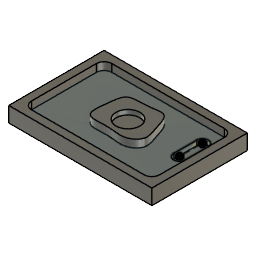
Cam Milling 1 (Autodesk Fusion 360 design; units mm, degrees)
part number: 2026-06-20-21-11-02-857
Autodesk Fusion 360 part; units mm, degrees
sketch "Sketch1" plane through (0, 0, 0) normal (0, 0, 1) x (1, 0, 0)
  line L0 (-75, 50) -> (75, 50)
  line L1 (75, 50) -> (75, -50)
  line L2 (75, -50) -> (-75, -50)
  line L3 (-75, -50) -> (-75, 50)
  line L4 (-75, 50) -> (75, -50) construction
  line L5 (75, 50) -> (-75, -50) construction
  line L6 (59, -42) -> (-59, -42)
  line L7 (-67, -34) -> (-67, 34)
  line L8 (-59, 42) -> (59, 42)
  line L9 (67, 34) -> (67, -34)
  spline S0 degree 5 poles (0, 22.4638) (-0.8512, 22.3723) (-2.5749, 22.2065) (-5.2041, 22.0186) (-8.7034, 21.8851) (-12.8111, 21.7572) (-16.4137, 21.4266) (-19.3328, 20.6302) (-21.4856, 19.1397) (-22.9396, 16.8333) (-23.8797, 13.7066) (-24.5296, 9.8513) (-25.0848, 5.4458) (-25.6462, 0.739) (-26.1388, -3.9587) (-26.3602, -8.3171) (-26.0551, -12.0321) (-24.9834, -14.8737) (-22.9846, -16.7269) (-20.0608, -17.6506) (-16.39, -17.8744) (-12.2425, -17.7077) (-7.9213, -17.4694) (-3.6953, -17.4135) (0.2717, -17.6471) (3.9677, -18.0777) (7.463, -18.4971) (10.8553, -18.6466) (14.2107, -18.2888) (17.5046, -17.2781) (20.5668, -15.6275) (23.1569, -13.4486) (25.0395, -10.8925) (26.0506, -8.0979) (26.1887, -5.1193) (25.6129, -1.9281) (24.5591, 1.5242) (23.2765, 5.2568) (21.9612, 9.2114) (20.6767, 13.1862) (19.3688, 16.8808) (17.9149, 19.9787) (16.1624, 22.2215) (13.9692, 23.4772) (11.2494, 23.8354) (7.9839, 23.5599) (4.97, 23.0978) (2.5324, 22.7554) (0.8512, 22.5553) (0, 22.4638) knots 0 0 0 0 0 0 0.022222 0.044444 0.066667 0.088889 0.111111 0.133333 0.155556 0.177778 0.2 0.222222 0.244444 0.266667 0.288889 0.311111 0.333333 0.355556 0.377778 0.4 0.422222 0.444444 0.466667 0.488889 0.511111 0.533333 0.555556 0.577778 0.6 0.622222 0.644444 0.666667 0.688889 0.711111 0.733333 0.755556 0.777778 0.8 0.822222 0.844444 0.866667 0.888889 0.911111 0.933333 0.955556 0.977778 1 1 1 1 1 1
  arc A0 (-59, 42) -> (-67, 34) centre (-59, 34) ccw
  arc A1 (67, 34) -> (59, 42) centre (59, 34) ccw
  arc A2 (59, -42) -> (67, -34) centre (59, -34) ccw
  arc A3 (-67, -34) -> (-59, -42) centre (-59, -34) ccw
  point P0 (-20, 20)
  point P1 (-25.1867, 4.5381)
  point P2 (-23.7205, -15.8137)
  point P3 (-4.5381, -17.4719)
  point P4 (14.0682, -18.1526)
  point P5 (25.4136, -9.5301)
  point P6 (22.9176, 6.3534)
  point P7 (15.4297, 22.4638)
  dimension "d1" = 100
  dimension "d2" = 150
  dimension "d9" = 8
  constraint horizontal L0
  constraint perpendicular L0 L1
  constraint parallel L0 L2
  constraint parallel L1 L3
  constraint coincident L4 origin
  constraint coincident L5 origin
  constraint coincident L5 P2
  constraint tangent L7 A0
  constraint tangent L8 A0
  constraint tangent L8 A1
  constraint tangent L9 A1
  constraint equal A0 A1
  constraint tangent L6 A2
  constraint tangent L9 A2
  constraint equal A0 A2
  constraint tangent L6 A3
  constraint tangent L7 A3
  constraint equal A0 A3
  measures "d1" distance of L0.end L1.end
  measures "d2" distance of L1 L3
  measures "d9" radius of A0
extrude "Extrude1" add sketch "Sketch1" along normal blind 8 contours L0 L1 L2 L3 | L6 L7 L8 L9 A0 A1 A2 A3 | S0 makes body 1
extrude "Extrude2" add sketch "Sketch1" along normal blind 8 from surface at 8 bodies 1
sketch "Sketch2" plane through (0, 0, 8) normal (0, 0, 1) x (-1, 0, 0)
  spline S0 degree 5 poles (0, -22.4638) (-0.8512, -22.5553) (-2.5324, -22.7554) (-4.97, -23.0978) (-7.9839, -23.5599) (-11.2494, -23.8354) (-13.9692, -23.4772) (-16.1624, -22.2215) (-17.9149, -19.9787) (-19.3688, -16.8808) (-20.6767, -13.1862) (-21.9612, -9.2114) (-23.2765, -5.2568) (-24.5591, -1.5242) (-25.6129, 1.9281) (-26.1887, 5.1193) (-26.0506, 8.0979) (-25.0395, 10.8925) (-23.1569, 13.4486) (-20.5668, 15.6275) (-17.5046, 17.2781) (-14.2107, 18.2888) (-10.8553, 18.6466) (-7.463, 18.4971) (-3.9677, 18.0777) (-0.2717, 17.6471) (3.6953, 17.4135) (7.9213, 17.4694) (12.2425, 17.7077) (16.39, 17.8744) (20.0608, 17.6506) (22.9846, 16.7269) (24.9834, 14.8737) (26.0551, 12.0321) (26.3602, 8.3171) (26.1388, 3.9587) (25.6462, -0.739) (25.0848, -5.4458) (24.5296, -9.8513) (23.8797, -13.7066) (22.9396, -16.8333) (21.4856, -19.1397) (19.3328, -20.6302) (16.4137, -21.4266) (12.8111, -21.7572) (8.7034, -21.8851) (5.2041, -22.0186) (2.5749, -22.2065) (0.8512, -22.3723) (0, -22.4638) knots -1 -1 -1 -1 -1 -1 -0.977778 -0.955556 -0.933333 -0.911111 -0.888889 -0.866667 -0.844444 -0.822222 -0.8 -0.777778 -0.755556 -0.733333 -0.711111 -0.688889 -0.666667 -0.644444 -0.622222 -0.6 -0.577778 -0.555556 -0.533333 -0.511111 -0.488889 -0.466667 -0.444444 -0.422222 -0.4 -0.377778 -0.355556 -0.333333 -0.311111 -0.288889 -0.266667 -0.244444 -0.222222 -0.2 -0.177778 -0.155556 -0.133333 -0.111111 -0.088889 -0.066667 -0.044444 -0.022222 0 0 0 0 0 0
  line L0 (67, -34) -> (67, 34)
  arc A0 (67, 34) -> (59, 42) centre (59, 34) ccw
  line L1 (59, 42) -> (-59, 42)
  arc A1 (-59, 42) -> (-67, 34) centre (-59, 34) ccw
  line L2 (-67, 34) -> (-67, -34)
  arc A2 (-67, -34) -> (-59, -42) centre (-59, -34) ccw
  line L3 (-59, -42) -> (59, -42)
  arc A3 (59, -42) -> (67, -34) centre (59, -34) ccw
  line L4 (-47, -25) -> (-47, -1)
  arc A4 (-47, -1) -> (-59, -1) centre (-53, -1) ccw
  line L5 (-59, -1) -> (-59, -25)
  arc A5 (-59, -25) -> (-47, -25) centre (-53, -25) ccw
  line L6 (-53, -25) -> (-53, -1) construction
  dimension "d10" = 24
  dimension "d11" = 6
  dimension "d12" = 14
  dimension "d13" = 17
  constraint tangent L4 A4
  constraint tangent A4 L5
  constraint parallel L4 L5
  constraint tangent L5 A5
  constraint tangent L4 A5
  constraint vertical L6
  measures "d10" distance of A5.centre A4.centre
  measures "d11" radius of A5
  measures "d12" distance of L2 L6
  measures "d13" distance of L3 A5.centre
surface "Extrude3" add extruded along (0, 0, 1) between 0 and -8 profiles "Sketch2" section 1 contours L4 A4 L5 A5 separate body makes body 2
extrude "Extrude4" cut sketch "Sketch2" against normal blind 5 contours L4 A4 L5 A5 bodies 1
sketch "Sketch3" plane through (0, 0, 16) normal (0, 0, 1) x (-1, 0, 0)
  spline S0 degree 5 poles (0, -22.4638) (0.8512, -22.3723) (2.5749, -22.2065) (5.2041, -22.0186) (8.7034, -21.8851) (12.8111, -21.7572) (16.4137, -21.4266) (19.3328, -20.6302) (21.4856, -19.1397) (22.9396, -16.8333) (23.8797, -13.7066) (24.5296, -9.8513) (25.0848, -5.4458) (25.6462, -0.739) (26.1388, 3.9587) (26.3602, 8.3171) (26.0551, 12.0321) (24.9834, 14.8737) (22.9846, 16.7269) (20.0608, 17.6506) (16.39, 17.8744) (12.2425, 17.7077) (7.9213, 17.4694) (3.6953, 17.4135) (-0.2717, 17.6471) (-3.9677, 18.0777) (-7.463, 18.4971) (-10.8553, 18.6466) (-14.2107, 18.2888) (-17.5046, 17.2781) (-20.5668, 15.6275) (-23.1569, 13.4486) (-25.0395, 10.8925) (-26.0506, 8.0979) (-26.1887, 5.1193) (-25.6129, 1.9281) (-24.5591, -1.5242) (-23.2765, -5.2568) (-21.9612, -9.2114) (-20.6767, -13.1862) (-19.3688, -16.8808) (-17.9149, -19.9787) (-16.1624, -22.2215) (-13.9692, -23.4772) (-11.2494, -23.8354) (-7.9839, -23.5599) (-4.97, -23.0978) (-2.5324, -22.7554) (-0.8512, -22.5553) (0, -22.4638) knots 0 0 0 0 0 0 0.022222 0.044444 0.066667 0.088889 0.111111 0.133333 0.155556 0.177778 0.2 0.222222 0.244444 0.266667 0.288889 0.311111 0.333333 0.355556 0.377778 0.4 0.422222 0.444444 0.466667 0.488889 0.511111 0.533333 0.555556 0.577778 0.6 0.622222 0.644444 0.666667 0.688889 0.711111 0.733333 0.755556 0.777778 0.8 0.822222 0.844444 0.866667 0.888889 0.911111 0.933333 0.955556 0.977778 1 1 1 1 1 1
  circle A0 centre (0, 0) radius 12.5
  dimension "d18" = 25
  constraint coincident A0.centre origin
  measures "d18" diameter of A0
extrude "Extrude5" cut sketch "Sketch3" against normal blind 5 contours A0 bodies 1
